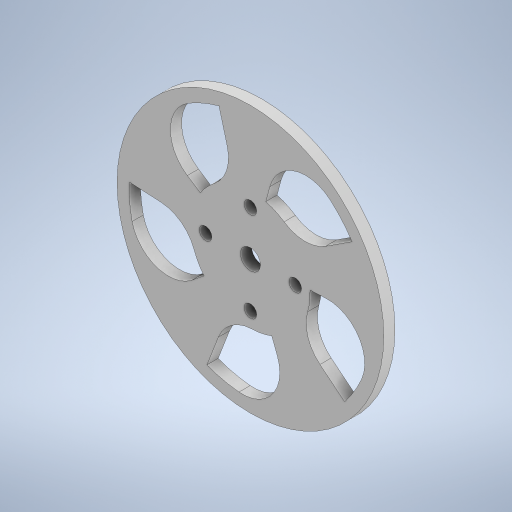
# Autodesk Inventor part: Wheel_2D_Int
Saved by Autodesk Inventor 2023 (Build 270158000, 158)
## iProperties
Created: 2024-08-05
Part Number: Wheel_2D_Int
Material: Generic
Document SubType Name: Modeling
Designer: LEGION
Density: 1 g/cm^3
Appearance: Default
Author: LEGION
Autodesk Inventor part; units mm, degrees
ref_plane "YZ Plane" through (0, 0, 0) normal (1, 0, 0) x (0, 1, 0)
ref_plane "XZ Plane" through (0, 0, 0) normal (0, 1, 0) x (-1, 0, 0)
ref_plane "XY Plane" through (0, 0, 0) normal (0, 0, 1) x (1, 0, 0)
sketch "Sketch1" plane through (0, 0, 0) normal (0, 0, 1) x (1, 0, 0)
  circle A0 centre (0, 0) radius 35.75
  circle A1 centre (0, 0) radius 32.5
  circle A2 centre (0, 0) radius 16
  circle A3 centre (0, 0) radius 2.7
  line L0 (0, 0) -> (-8.4116, 31.3926)
  line L1 (0, 0) -> (8.4116, 31.3926)
  line L2 (0, 0) -> (0, 4.5704)
  line L3 (0, 0) -> (-32.4555, 1.7009)
  line L4 (0, 0) -> (-27.2568, 17.7008)
  line L5 (0, 0) -> (-11.647, -30.3414)
  line L6 (0, 0) -> (-25.2572, -20.4529)
  line L7 (0, 0) -> (25.2572, -20.4529)
  line L8 (0, 0) -> (11.647, -30.3414)
  line L9 (0, 0) -> (27.2568, 17.7008)
  line L10 (0, 0) -> (32.4555, 1.7009)
  point P0 (4.1411, 15.4548)
  point P1 (13.4187, 8.7142)
  point P2 (-4.1411, 15.4548)
  point P3 (-13.4187, 8.7142)
  point P4 (12.4343, -10.0691)
  point P5 (15.9781, 0.8374)
  point P6 (-5.7339, -14.9373)
  point P7 (5.7339, -14.9373)
  point P8 (-15.9781, 0.8374)
  point P9 (-12.4343, -10.0691)
  dimension "d0" = 71.5
  dimension "d1" = 65
  dimension "d2" = 5.4
  dimension "d3" = 32
  dimension "d4" = 15
  dimension "d5" = 15
  dimension "d8" = 360
  constraints: 22 end point, 4 centre point, 4 coincident, 2 point on circle, 1 vertical, 26 other
  measures "d0" diameter of A0
  measures "d1" diameter of A1
  measures "d2" diameter of A3
  measures "d3" diameter of A2
  measures "d4" angle of L1 L2
  measures "d5" angle of L2 L0
extrude "Extrusion1" add sketch "Sketch1" along normal blind 3 contours A0 | L10 A2 L9 A1 | A1 L8 A2 L7 | L10 A3 L9 A2 | A2 L7 A3 L10 | A2 L8 A3 L7 | L1 A2 L0 A1 | L9 A3 L1 A2 | A1 L6 A2 L5 | A2 L5 A3 L8 | L1 A3 L0 A2 | A2 L6 A3 L5 | L4 A2 L3 A1 | L0 A3 L4 A2 | L3 A2 L4 A3 | A3 L6 A2 L3
fillet "Fillet1" radius 10 10 edges at (8.4116, 31.3926, 1.5) (-27.2568, 17.7008, 1.5) (-25.2572, -20.4529, 1.5) (11.647, -30.3414, 1.5) (32.4555, 1.7009, 1.5) (-15.9781, 0.8374, 1.5) (-4.1411, 15.4548, 1.5) (13.4187, 8.7142, 1.5) (12.4343, -10.0691, 1.5) (-5.7339, -14.9373, 1.5)
sketch "Sketch2" plane through (0, 0, 3) normal (0, 0, 1) x (1, 0, 0)
  circle A0 centre (0, 12.0208) radius 1.7
  circle A1 centre (-12.0208, 0) radius 1.7
  circle A2 centre (0, -12.0208) radius 1.7
  circle A3 centre (12.0208, 0) radius 1.7
  line L0 (0, 12.0208) -> (-12.0208, 0)
  line L1 (-12.0208, 0) -> (0, -12.0208)
  line L2 (0, -12.0208) -> (12.0208, 0)
  line L3 (12.0208, 0) -> (0, 12.0208)
  point P0 (0, 0)
  dimension "d13" = 17
  dimension "d14" = 17
  dimension "d15" = 3.4
  dimension "d16" = 3.4
  dimension "d17" = 3.4
  dimension "d18" = 3.4
  constraints: 8 end point, 4 centre point, 2 horizontal alignment, 2 perpendicular, 1 parallel, 1 vertical alignment
  measures "d13" distance of L1.end L2.end
  measures "d14" distance of L2.end L0.start
  measures "d15" diameter of A3
  measures "d16" diameter of A2
  measures "d17" diameter of A0
  measures "d18" diameter of A1
extrude "Extrusion2" cut sketch "Sketch2" against normal blind 3 contours A0 L3 L0 | L0 L3 A0 | L0 L1 A1 | A1 L1 L0 | L3 L2 A3 | A3 L2 L3 | L1 L2 A2 | A2 L2 L1
body "Solid1"
